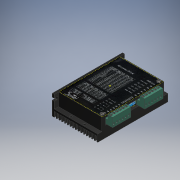
# Autodesk Inventor part: Microstep Driver
Saved by Autodesk Inventor 2017 SP1 (Build 210196100, 196)
## iProperties
Created: 2017-06-12
Part Number: Microstep Driver
Material: Generic
Document SubType Name: Modeling
Designer: sergo
Density: 1 g/cm^3
Appearance: Glossy - Black
Author: sergo
Autodesk Inventor part; units mm, degrees
ref_plane "YZ Plane" through (0, 0, 0) normal (1, 0, 0) x (0, 1, 0)
ref_plane "XZ Plane" through (0, 0, 0) normal (0, 1, 0) x (-1, 0, 0)
ref_plane "XY Plane" through (0, 0, 0) normal (0, 0, 1) x (1, 0, 0)
sketch "Sketch1" plane through (0, 0, 0) normal (0, 0, 1) x (1, 0, 0)
  line L0 (-58.75, -38) -> (58.75, -38)
  line L1 (58.75, -38) -> (58.75, 38)
  line L2 (58.75, 38) -> (-58.75, 38)
  line L3 (-58.75, 38) -> (-58.75, -38)
  line L4 (-58.75, -38) -> (58.75, 38) construction
  line L5 (58.75, -38) -> (-58.75, 38) construction
  point P0 (0, 0)
  dimension "d0" = 117.5
  dimension "d1" = 76
  constraints: 12 end point, 2 midpoint, 2 parallel, 1 horizontal, 1 perpendicular
  measures "d0" distance of L2.end L1.end
  measures "d1" distance of L1.end L0.end
extrude "Extrusion1" add sketch "Sketch1" along normal blind 33
sketch "Sketch2" plane through (58.75, -38, 0) normal (1, 0, 0) x (0, 0, -1)
  line L0 (0, 3.5) -> (-8.5, 3.5)
  line L1 (-8.5, 3.5) -> (-8.5, 6.7)
  line L2 (-8.5, 6.7) -> (0, 6.7)
  line L3 (0, 6.7) -> (0, 3.5)
  point P0 (0, 38)
  point P1 (0, 0)
  point P2 (0, 5.1)
  dimension "d4" = 8.5
  dimension "d5" = 3.2
  dimension "d6" = 3.5
  constraints: 8 end point, 2 parallel, 1 horizontal, 1 midpoint, 1 perpendicular, 1 vertical alignment
  measures "d4" distance of L1.end L2.end
  measures "d5" distance of L0.end L1.end
  measures "d6" distance of point (0, 0) L0.start
extrude "Extrusion2" cut sketch "Sketch2" against normal through all
pattern_linear "Rectangular Pattern1" count 16 spacing 4.54 along (0, 1, 0) of "Extrusion2"
sketch "Sketch3" plane through (0, 0, 33) normal (0, 0, 1) x (1, 0, 0)
  line L0 (58.75, -38) -> (58.75, 38) projected
  line L1 (58.75, 38) -> (-58.75, 38) projected
  line L2 (58.75, -34.5) -> (51.55, -34.5)
  line L3 (51.55, -34.5) -> (51.55, 38)
  line L4 (51.55, 38) -> (58.75, 38)
  line L5 (58.75, 38) -> (58.75, -34.5)
  point P0 (0, 0)
  point P1 (-58.75, -38)
  dimension "d12" = 3.5
  dimension "d13" = 7.2
  constraints: 8 end point, 2 parallel, 2 point on line, 1 horizontal, 1 perpendicular
  measures "d12" distance of L0.start L2.start
  measures "d13" distance of L2.start L2.end
extrude "Extrusion3" cut sketch "Sketch3" against normal blind 21.1
mirror "Mirror1" about plane through (0, 0, 0) normal (1, 0, 0) of "Extrusion3"
sketch "Sketch4" plane through (0, 0, 33) normal (0, 0, 1) x (1, 0, 0)
  line L0 (-50.6807, -34.4871) -> (-50.6807, 37.9875) construction
  line L1 (-50.6807, 37.9875) -> (50.75, 37.9875) construction
  line L2 (50.75, 37.9875) -> (50.75, -34.4871) construction
  line L3 (50.75, -34.4871) -> (-50.6807, -34.4871) construction
  point P0 (0, 0)
  constraints: 2 other
sketch "Sketch5" plane through (0, 0, 11.9) normal (0, 0, 1) x (1, 0, 0)
  point P0 (0, 0)
  point P1 (55.5, -10)
  point P2 (55.5, 12.5)
  point P3 (-55.5, 12.5)
  point P4 (-55.5, -10)
  point P5 (58.75, -38)
  dimension "d22" = 111
  dimension "d23" = 55.5
  dimension "d24" = 28
  dimension "d25" = 22.5
  constraints: 2 horizontal alignment, 2 vertical alignment
  measures "d22" distance of point (55.5, 12.5) point (-55.5, 12.5)
  measures "d23" horizontal distance of point (0, 0) point (-55.5, 12.5)
  measures "d24" vertical distance of point (58.75, -38) point (55.5, -10)
  measures "d25" distance of point (55.5, -10) point (55.5, 12.5)
hole "Hole1" at (55.5, 12.5, 11.9) at (55.5, -10, 11.9) at (-55.5, -10, 11.9) at (-55.5, 12.5, 11.9) direction (0, 0, -1) diameter 3.2 end through all
sketch "Sketch6" plane through (-58.75, 38, 0) normal (0, 1, 0) x (1, 0, 0)
  line L0 (7.2, -11.9) -> (7.2, -33) projected
  line L1 (110.3, -33) -> (7.2, -33) projected
  line L2 (110.3, -33) -> (110.3, -11.9) projected
  line L3 (110.3, -11.9) -> (117.5, -11.9) projected
  line L4 (117.5, 0) -> (117.5, -11.9) projected
  line L5 (117.5, 0) -> (0, 0) projected
  line L6 (0, 0) -> (0, -11.9) projected
  line L7 (0, -11.9) -> (7.2, -11.9) projected
  line L8 (104.25, -29) -> (13.25, -29)
  line L9 (13.25, -29) -> (13.25, -18.3)
  line L10 (13.25, -18.3) -> (104.25, -18.3)
  line L11 (104.25, -18.3) -> (104.25, -29)
  line L12 (117.5, 0) -> (0, 0) projected
  point P0 (58.75, 0)
  point P1 (58.75, -18.3)
  point P2 (58.75, 0)
  dimension "d35" = 91
  dimension "d36" = 4
  dimension "d37" = 10.7
  constraints: 8 end point, 2 midpoint, 2 parallel, 1 horizontal, 1 perpendicular, 1 vertical alignment
  measures "d35" distance of L8.start L8.end
  measures "d36" distance between parallel lines of L8 L1
  measures "d37" distance between parallel lines of L10 L8
extrude "Extrusion4" cut sketch "Sketch6" against normal blind 3.7 contours L8 L9 L10 L11
sketch "Sketch7" plane through (-58.75, 34.3, 0) normal (0, 1, 0) x (1, 0, 0)
  line L0 (104.25, -29) -> (13.25, -29) projected
  line L1 (104.25, -18.3) -> (104.25, -29) projected
  line L2 (13.25, -18.3) -> (104.25, -18.3) projected
  line L3 (13.25, -29) -> (13.25, -18.3) projected
  line L4 (104.25, -29) -> (13.25, -29) projected
  line L5 (71.9, -26.3) -> (71.9, -18.6)
  line L6 (71.9, -18.6) -> (102.5, -18.6)
  line L7 (102.5, -18.6) -> (102.5, -26.3)
  line L8 (48.9, -26.3) -> (48.9, -18.6)
  line L9 (48.9, -18.6) -> (18.3, -18.6)
  line L10 (18.3, -18.6) -> (18.3, -26.3)
  line L11 (102.5, -26.3) -> (71.9, -26.3)
  line L12 (48.9, -26.3) -> (18.3, -26.3)
  point P0 (58.75, 0)
  point P1 (117.5, -8.5)
  dimension "d40" = 30.6
  dimension "d41" = 23
  dimension "d42" = 30.6
  dimension "d43" = 0.3
  dimension "d44" = 7.7
  dimension "d45" = 15
  constraints: 16 end point, 2 collinear, 2 parallel, 2 perpendicular, 1 point on line
  measures "d40" distance of L5.end L6.end
  measures "d41" distance between parallel lines of L8 L5
  measures "d42" distance between parallel lines of L10 L8
  measures "d43" distance between parallel lines of L2 L6
  measures "d44" distance between parallel lines of L11 L6
  measures "d45" distance from line of point (117.5, -8.5) L7
extrude "Extrusion5" add sketch "Sketch7" along normal blind 5.7 contours L5 L6 L7 L11 | L12 L10 L9 L8
sketch "Sketch8" plane through (-58.75, 40, 0) normal (0, 1, 0) x (1, 0, 0)
  line L0 (71.9, -18.6) -> (71.9, -26.3) projected
  line L1 (71.9, -26.3) -> (102.5, -26.3) projected
  line L2 (102.5, -26.3) -> (102.5, -18.6) projected
  line L3 (102.5, -18.6) -> (71.9, -18.6) projected
  line L4 (18.3, -18.6) -> (18.3, -26.3) projected
  line L5 (18.3, -26.3) -> (48.9, -26.3) projected
  line L6 (48.9, -26.3) -> (48.9, -18.6) projected
  line L7 (48.9, -18.6) -> (18.3, -18.6) projected
  line L8 (102.5, -18.6) -> (71.9, -18.6)
  line L9 (71.9, -18.6) -> (71.9, -33.7)
  line L10 (71.9, -33.7) -> (102.5, -33.7)
  line L11 (102.5, -33.7) -> (102.5, -18.6)
  line L12 (48.9, -18.6) -> (18.3, -18.6)
  line L13 (18.3, -18.6) -> (18.3, -33.7)
  line L14 (18.3, -33.7) -> (48.9, -33.7)
  line L15 (48.9, -33.7) -> (48.9, -18.6)
  line L16 (71.9, -18.6) -> (71.9, -26.3) projected
  line L17 (18.3, -18.6) -> (18.3, -26.3) projected
  point P0 (58.75, 0)
  dimension "d48" = 15.1
  constraints: 16 end point, 4 parallel, 3 collinear, 2 horizontal, 2 perpendicular
  measures "d48" distance between parallel lines of L10 L3
extrude "Extrusion6" add sketch "Sketch8" along normal blind 8
sketch "Sketch10" plane through (-58.75, 48, 0) normal (0, 1, 0) x (1, 0, 0)
  line L0 (102.5, -18.6) -> (71.9, -18.6) projected
  line L1 (71.9, -18.6) -> (71.9, -33.7) projected
  line L2 (71.9, -33.7) -> (102.5, -33.7) projected
  line L3 (102.5, -33.7) -> (102.5, -18.6) projected
  line L4 (48.9, -18.6) -> (18.3, -18.6) projected
  line L5 (18.3, -18.6) -> (18.3, -33.7) projected
  line L6 (18.3, -33.7) -> (48.9, -33.7) projected
  line L7 (48.9, -33.7) -> (48.9, -18.6) projected
  line L8 (101.5, -21.6) -> (98.8, -21.6)
  line L9 (98.8, -21.6) -> (98.8, -25.3)
  line L10 (98.8, -25.3) -> (101.5, -25.3)
  line L11 (101.5, -25.3) -> (101.5, -21.6)
  point P0 (58.75, 0)
  dimension "d51" = 2.7
  dimension "d52" = 3.7
  dimension "d53" = 1
  dimension "d54" = 3
  constraints: 8 end point, 2 parallel, 1 horizontal, 1 perpendicular
  measures "d51" distance of L10.end L9.end
  measures "d52" distance of L9.end L8.end
  measures "d53" distance between parallel lines of L3 L11
  measures "d54" distance between parallel lines of L0 L8
extrude "Extrusion7" cut sketch "Sketch10" against normal blind 7 contours L11 L10 L9 L8
pattern_linear "Rectangular Pattern2" count 6 spacing 5 along (-1, 0, 0) of "Extrusion7"
pattern_linear "Rectangular Pattern3" count 2 spacing 53.7 along (-1, 0, 0) of "Extrusion7", "Rectangular Pattern2"
sketch "Sketch11" plane through (0, 0, 33) normal (0, 0, 1) x (1, 0, 0)
  circle A0 centre (47.35, 34) radius 2.75
  circle A1 centre (-47.35, 34) radius 2.75
  line L0 (-51.55, 38) -> (-51.55, -34.5) projected
  line L1 (51.55, -34.5) -> (51.55, 38) projected
  line L2 (51.55, 38) -> (-51.55, 38) projected
  point P0 (0, 0)
  dimension "d65" = 5.5
  dimension "d66" = 5.5
  dimension "d67" = 4.2
  dimension "d68" = 4.2
  dimension "d69" = 4
  constraints: 2 centre point, 1 horizontal alignment
  measures "d65" diameter of A0
  measures "d66" diameter of A1
  measures "d67" distance from line of A1.centre L0
  measures "d68" distance from line of A0.centre L1
  measures "d69" distance from line of L2 A1.centre
extrude "Extrusion8" add sketch "Sketch11" along normal blind 2
fillet "Fillet1" radius 0.9 2 edges at (44.6, 34, 35) (-50.1, 34, 35)
sketch "Sketch12" plane through (47.35, 34, 35) normal (0, 0, 1) x (1, 0, 0)
  line L0 (3, -0.4) -> (-3, -0.4)
  line L1 (-3, -0.4) -> (-3, 0.4)
  line L2 (-3, 0.4) -> (3, 0.4)
  line L3 (3, 0.4) -> (3, -0.4)
  point P0 (-47.35, -34)
  point P1 (3, 0)
  point P2 (0, 0.4)
  dimension "d72" = 0.8
  dimension "d73" = 6
  constraints: 8 end point, 2 midpoint, 2 parallel, 1 horizontal, 1 perpendicular
  measures "d72" distance between parallel lines of L2 L0
  measures "d73" distance of L0.start L0.end
extrude "Extrusion9" cut sketch "Sketch12" against normal blind 1
mirror "Mirror2" about plane through (0, 0, 0) normal (1, 0, 0) of "Extrusion9"
sketch "Sketch13" plane through (-58.75, 34.3, 0) normal (0, 1, 0) x (1, 0, 0)
  circle A0 centre (15.7473, -26.3809) radius 1.5
  circle A1 centre (15.7473, -21.9403) radius 1.5
  point P0 (58.75, 0)
  dimension "d77" = 3
  dimension "d78" = 3
  constraints: 2 centre point, 1 vertical alignment
  measures "d77" diameter of A0
  measures "d78" diameter of A1
extrude "Extrusion10" add sketch "Sketch13" along normal blind 4
fillet "Fillet2" radius 1.5 2 edges at (-44.5027, 38.3, 26.3809) (-44.5027, 38.3, 21.9403)
sketch "Sketch14" plane through (-58.75, 34.3, 0) normal (0, 1, 0) x (1, 0, 0)
  line L0 (70.5606, -28.1681) -> (49.9748, -28.1681) construction
  line L1 (49.9748, -28.1681) -> (49.9748, -19.2668) construction
  line L2 (49.9748, -19.2668) -> (70.5606, -19.2668) construction
  line L3 (70.5606, -19.2668) -> (70.5606, -28.1681) construction
  point P0 (58.75, 0)
  constraints: 2 other
sketch "Sketch15" plane through (13.15, 40, 33.7) normal (0, 0, 1) x (1, 0, 0)
  line L0 (29.6, 8) -> (26.9, 8) projected
  line L1 (24.6, 8) -> (21.9, 8) projected
  line L2 (19.6, 8) -> (16.9, 8) projected
  line L3 (14.6, 8) -> (11.9, 8) projected
  line L4 (9.6, 8) -> (6.9, 8) projected
  line L5 (4.6, 8) -> (1.9, 8) projected
  line L6 (-24.1, 8) -> (-26.8, 8) projected
  line L7 (-29.1, 8) -> (-31.8, 8) projected
  line L8 (-34.1, 8) -> (-36.8, 8) projected
  line L9 (-39.1, 8) -> (-41.8, 8) projected
  line L10 (-44.1, 8) -> (-46.8, 8) projected
  line L11 (-49.1, 8) -> (-51.8, 8) projected
  point P0 (-13.15, -40)
  point P1 (28.25, 2.8)
  point P2 (23.25, 2.8)
  point P3 (18.25, 2.8)
  point P4 (13.25, 2.8)
  point P5 (8.25, 2.8)
  point P6 (3.25, 2.8)
  point P7 (-25.45, 2.8)
  point P8 (-30.45, 2.8)
  point P9 (-35.45, 2.8)
  point P10 (-40.45, 2.8)
  point P11 (-45.45, 2.8)
  point P12 (-50.45, 2.8)
  point P13 (28.25, 8)
  point P14 (23.25, 8)
  point P15 (18.25, 8)
  point P16 (13.25, 8)
  point P17 (8.25, 8)
  point P18 (3.25, 8)
  point P19 (-25.45, 8)
  point P20 (-30.45, 8)
  point P21 (-35.45, 8)
  point P22 (-40.45, 8)
  point P23 (-45.45, 8)
  point P24 (-50.45, 8)
  dimension "d103" = 5.2
  constraints: 12 midpoint, 12 vertical alignment, 11 horizontal alignment
  measures "d103" distance from line of L0 point (28.25, 2.8)
hole "Hole2" at (-37.3, 42.8, 33.7) at (-32.3, 42.8, 33.7) at (-27.3, 42.8, 33.7) at (-22.3, 42.8, 33.7) at (-17.3, 42.8, 33.7) at (-12.3, 42.8, 33.7) at (16.4, 42.8, 33.7) at (21.4, 42.8, 33.7) at (26.4, 42.8, 33.7) at (31.4, 42.8, 33.7) at (36.4, 42.8, 33.7) at (41.4, 42.8, 33.7) direction (0, 0, -1) diameter 4 depth 1
sketch "Sketch16" plane through (41.4, 42.8, 32.7) normal (0, 0, 1) x (1, 0, 0)
  line L0 (1.96, -0.3981) -> (-1.96, -0.3981)
  line L1 (-1.9592, 0.4019) -> (1.9592, 0.4019)
  circle A0 centre (0, 0) radius 2 construction
  circle A1 centre (0, 0) radius 2 construction
  arc A2 (1.9595, -0.4002) -> (1.9588, 0.4037) centre (0, 0) ccw
  arc A3 (-1.9592, 0.4019) -> (-1.96, -0.3981) centre (0, 0) ccw
  point P0 (-41.4, -42.8)
  point P1 (0, 0.4019)
  point P2 (1.9592, 0.4019)
  dimension "d111" = 0.8
  constraints: 15 point on circle, 4 end point, 2 centre point, 1 horizontal, 1 midpoint, 1 parallel, 1 point on line, 1 vertical alignment
  measures "d111" distance between parallel lines of L1 L0
extrude "Extrusion11" cut sketch "Sketch16" against normal blind 0.8
pattern_linear "Rectangular Pattern4" count 6 spacing 5 along (-1, 0, 0) of "Extrusion11"
pattern_linear "Rectangular Pattern5" count 2 spacing 53.7 along (-1, 0, 0) of "Extrusion11", "Rectangular Pattern4"
sketch "Sketch17" plane through (-58.75, -34.5, 33) normal (0, 1, 0) x (1, 0, 0)
  line L0 (4, 5.6) -> (0, 5.6)
  line L1 (0, 5.6) -> (0, 9.8)
  line L2 (0, 9.8) -> (4, 9.8)
  arc A0 (4, 5.6) -> (4, 9.8) centre (4, 7.7) ccw
  line L3 (0, 24.5) -> (0, 33) projected
  point P0 (58.75, 33)
  point P1 (0, 7.7)
  dimension "d121" = 4.2
  dimension "d122" = 23.2
  dimension "d123" = 4
  constraints: 6 end point, 2 point on circle, 1 centre point, 1 collinear, 1 horizontal, 1 horizontal alignment, 1 midpoint, 1 parallel, 1 perpendicular, 1 tangent
  measures "d121" distance between parallel lines of L2 L0
  measures "d122" distance from line of L2 L3.end
  measures "d123" horizontal distance of L3.end A0.centre
extrude "Extrusion12" cut sketch "Sketch17" against normal through all
mirror "Mirror3" about plane through (0, 0, 0) normal (1, 0, 0) of "Extrusion12"
chamfer "Chamfer1" distance 0.5 angle 45 4 edges at (-55.5, -8.4, 11.9) (-55.5, 14.1, 11.9) (55.5, -8.4, 11.9) (55.5, 14.1, 11.9)
equation "\"d23\" = 0.5 * d22"
body "Solid1"
